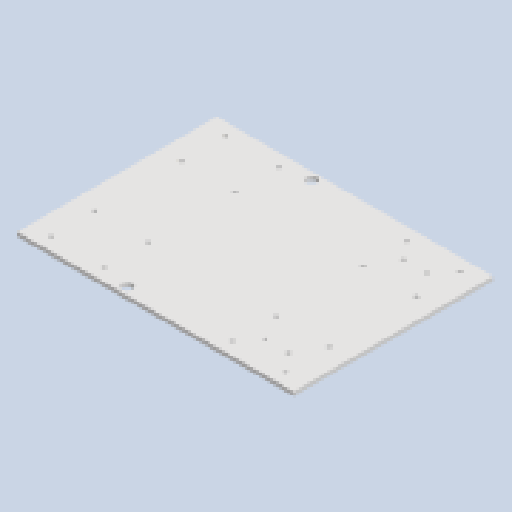
# Autodesk Inventor part: нижняя пластина
Saved by Autodesk Inventor 2024.2 (Build 282272000, 272)
## iProperties
Created: 2025-11-23
Part Number: нижняя пластина
Material: Типовые
Document SubType Name: Modeling
Designer: katya_notebook
Density: 1 g/cm^3
Appearance: По умолчанию
Author: katya_notebook
Autodesk Inventor part; units mm, degrees
ref_plane "YZ Plane" through (0, 0, 0) normal (1, 0, 0) x (0, 1, 0)
ref_plane "XZ Plane" through (0, 0, 0) normal (0, 1, 0) x (-1, 0, 0)
ref_plane "XY Plane" through (0, 0, 0) normal (0, 0, 1) x (1, 0, 0)
ref_plane "РабПлоскость1" through (-553.2789, -264.3002, 1.4222) normal (0, 1, 0) x (-1, 0, 0)
sketch "Эскиз1" plane through (-553.2789, -264.3002, 1.4222) normal (0, 1, 0) x (-1, 0, 0)
  line L0 (-30, 163.5) -> (30, 163.5) projected
  line L1 (-30, -31.5) -> (30, -31.5) projected
  line L2 (46.4763, 163.5) -> (-223.5237, 163.5)
  line L3 (-223.5237, 163.5) -> (-223.5237, -31.5)
  line L4 (-223.5237, -31.5) -> (46.4763, -31.5)
  line L5 (46.4763, -31.5) -> (46.4763, 163.5)
  point P0 (-553.2789, -1.4222)
  point P1 (-30, -30)
  point P2 (30, -30)
  point P3 (30, 162)
  point P4 (-30, 162)
  dimension "d1" = 270
  dimension "d6" = 0
  dimension "d7" = 0
  constraints: 8 end point, 2 coincident, 2 parallel, 1 horizontal, 1 perpendicular
  measures "d1" distance of L2.start L2.end
  measures "d6" distance from line of L4 L1.end
  measures "d7" distance from line of L2 L0.end
extrude "Выдавливание1" add sketch "Эскиз1" along normal blind 4
sketch "Эскиз2" plane through (-553.2789, -264.3002, 1.4222) normal (0, -1, 0) x (1, 0, 0)
  circle A0 centre (26, 108.5) radius 2 projected
  circle A1 centre (-26, 151) radius 2 projected
  circle A2 centre (26, 151) radius 2 projected
  circle A3 centre (-26, 108.5) radius 2 projected
  line L0 (-21.5, 122) -> (-21.5, 157) projected
  line L1 (-23.5, 122) -> (-21.5, 122) projected
  line L2 (-23.5, 157) -> (-23.5, 122) projected
  line L3 (-30, 157) -> (-23.5, 157) projected
  line L4 (-30, 157) -> (-30, 103.5) projected
  line L5 (-30, 103.5) -> (30, 103.5) projected
  line L6 (30, 103.5) -> (30, 157) projected
  line L7 (23.5, 157) -> (30, 157) projected
  line L8 (23.5, 122) -> (23.5, 157) projected
  line L9 (21.5, 122) -> (23.5, 122) projected
  line L10 (21.5, 157) -> (21.5, 122) projected
  line L11 (-21.5, 157) -> (21.5, 157) projected
  circle A4 centre (26, 23.5) radius 2 projected
  circle A5 centre (-26, -19) radius 2 projected
  circle A6 centre (26, -19) radius 2 projected
  circle A7 centre (-26, 23.5) radius 2 projected
  line L12 (-21.5, 10) -> (-21.5, -25) projected
  line L13 (-21.5, -25) -> (21.5, -25) projected
  line L14 (21.5, -25) -> (21.5, 10) projected
  line L15 (21.5, 10) -> (23.5, 10) projected
  line L16 (23.5, 10) -> (23.5, -25) projected
  line L17 (23.5, -25) -> (30, -25) projected
  line L18 (30, 28.5) -> (30, -25) projected
  line L19 (-30, 28.5) -> (30, 28.5) projected
  line L20 (-30, -25) -> (-30, 28.5) projected
  line L21 (-30, -25) -> (-23.5, -25) projected
  line L22 (-23.5, -25) -> (-23.5, 10) projected
  line L23 (-23.5, 10) -> (-21.5, 10) projected
  circle A8 centre (26, -19) radius 2
  circle A9 centre (26, 23.5) radius 2
  circle A10 centre (-26, -19) radius 2
  circle A11 centre (-26, 23.5) radius 2
  circle A12 centre (26, 108.5) radius 2
  circle A13 centre (26, 151) radius 2
  circle A14 centre (-26, 108.5) radius 2
  circle A15 centre (-26, 151) radius 2
  point P0 (553.2789, -1.4222)
  constraints: 8 centre point, 8 coincident, 8 concentric
extrude "Выдавливание2" cut sketch "Эскиз2" against normal blind 4 contours A0 | A1 | A2 | A3 | A4 | A5 | A6 | A7
sketch "Эскиз3" plane through (-553.2789, -264.3002, 1.4222) normal (0, -1, 0) x (1, 0, 0)
  spline S0 degree 3 poles (167.5306, -1.5) (167.5306, -1.6752) (167.5059, -1.8631) (167.407, -2.2163) (167.333, -2.3816) (167.1432, -2.702) (167.0026, -2.8694) (166.6948, -3.1391) (166.528, -3.2419) (165.9933, -3.4904) (165.5892, -3.534) (164.8487, -3.4171) (164.5121, -3.2574) (164.0242, -2.8457) (163.7999, -2.5683) (163.6284, -2.1264) (163.5929, -2.0111) (163.5438, -1.7621) (163.5306, -1.6279) (163.5306, -1.3721) (163.5438, -1.2379) (163.5929, -0.9889) (163.6284, -0.8736) (163.7999, -0.4317) (164.0242, -0.1543) (164.5121, 0.2574) (164.8487, 0.4171) (165.5892, 0.534) (165.9933, 0.4904) (166.528, 0.2419) (166.6948, 0.1391) (167.0026, -0.1306) (167.1432, -0.298) (167.333, -0.6184) (167.407, -0.7837) (167.5059, -1.1369) (167.5306, -1.3248) (167.5306, -1.5) knots -1.597181 -1.597181 -1.597181 -1.597181 -1.544613 -1.544613 -1.492044 -1.492044 -1.42258 -1.42258 -1.353115 -1.353115 -1.1824 -1.1824 -1.011685 -1.011685 -0.875329 -0.875329 -0.83696 -0.83696 -0.798591 -0.798591 -0.760221 -0.760221 -0.721852 -0.721852 -0.585496 -0.585496 -0.414781 -0.414781 -0.244066 -0.244066 -0.174601 -0.174601 -0.105137 -0.105137 -0.052568 -0.052568 0 0 0 0 projected
  spline S1 degree 3 poles (190.0475, -1.5) (190.0475, -1.6203) (190.0365, -1.7387) (189.9958, -1.9661) (189.9661, -2.0751) (189.8558, -2.3816) (189.7534, -2.5587) (189.3863, -3.0484) (189.0432, -3.2817) (188.267, -3.5292) (187.833, -3.5367) (187.2363, -3.3378) (187.0421, -3.2434) (186.6807, -2.9773) (186.5141, -2.805) (186.2864, -2.4643) (186.1972, -2.2855) (186.0776, -1.9002) (186.0475, -1.6935) (186.0475, -1.3065) (186.0776, -1.0998) (186.1972, -0.7145) (186.2864, -0.5357) (186.5141, -0.195) (186.6807, -0.0227) (187.0421, 0.2434) (187.2363, 0.3378) (187.833, 0.5367) (188.267, 0.5292) (189.0432, 0.2817) (189.3863, 0.0484) (189.7534, -0.4413) (189.8558, -0.6184) (189.9661, -0.9249) (189.9958, -1.0339) (190.0365, -1.2613) (190.0475, -1.3797) (190.0475, -1.5) knots -1.539921 -1.539921 -1.539921 -1.539921 -1.503835 -1.503835 -1.467748 -1.467748 -1.395575 -1.395575 -1.217174 -1.217174 -1.038772 -1.038772 -0.962412 -0.962412 -0.886052 -0.886052 -0.828007 -0.828007 -0.769961 -0.769961 -0.711915 -0.711915 -0.653869 -0.653869 -0.577509 -0.577509 -0.501149 -0.501149 -0.322747 -0.322747 -0.144346 -0.144346 -0.072173 -0.072173 -0.036086 -0.036086 0 0 0 0 projected
  circle A0 centre (203.0475, 23.5) radius 2 projected
  circle A1 centre (203.0475, -19) radius 2 projected
  circle A2 centre (151.0475, 23.5) radius 2 projected
  circle A3 centre (151.0475, -19) radius 2 projected
  line L0 (206.803, 28.5) -> (146.803, 28.5) projected
  line L1 (146.803, 28.5) -> (146.803, -25) projected
  line L2 (206.803, -25) -> (206.803, 28.5) projected
  line L3 (146.803, -25) -> (206.803, -25) projected
  point P0 (553.2789, -1.4222)
  point P1 (167.5306, -1.5)
  point P2 (190.0475, -1.5)
extrude "Выдавливание3" cut sketch "Эскиз3" against normal blind 10 contours S0 | S1 | A0 | A1 | A2 | A3
sketch "Эскиз4" plane through (-553.2789, -264.3002, 1.4222) normal (0, -1, 0) x (1, 0, 0)
  circle A0 centre (151.0475, 108.5) radius 2 projected
  circle A1 centre (203.0475, 108.5) radius 2 projected
  spline S0 degree 3 poles (190.0475, 133.5) (190.0475, 133.6203) (190.0365, 133.7387) (189.9958, 133.9661) (189.9661, 134.0751) (189.8558, 134.3816) (189.7534, 134.5587) (189.3863, 135.0484) (189.0432, 135.2817) (188.267, 135.5292) (187.833, 135.5367) (187.2363, 135.3378) (187.0421, 135.2435) (186.6807, 134.9773) (186.5141, 134.805) (186.2864, 134.4643) (186.1972, 134.2856) (186.0776, 133.9002) (186.0475, 133.6935) (186.0475, 133.3065) (186.0776, 133.0998) (186.1972, 132.7145) (186.2864, 132.5357) (186.5141, 132.195) (186.6807, 132.0227) (187.0421, 131.7566) (187.2363, 131.6622) (187.833, 131.4634) (188.267, 131.4708) (189.0432, 131.7183) (189.3863, 131.9517) (189.7534, 132.4413) (189.8558, 132.6184) (189.9661, 132.9249) (189.9958, 133.0339) (190.0365, 133.2613) (190.0475, 133.3797) (190.0475, 133.5) knots 0 0 0 0 0.036086 0.036086 0.072173 0.072173 0.144346 0.144346 0.322747 0.322747 0.501149 0.501149 0.577509 0.577509 0.653869 0.653869 0.711915 0.711915 0.769961 0.769961 0.828007 0.828007 0.886052 0.886052 0.962412 0.962412 1.038772 1.038772 1.217174 1.217174 1.395575 1.395575 1.467748 1.467748 1.503835 1.503835 1.539921 1.539921 1.539921 1.539921 projected
  spline S1 degree 3 poles (167.5306, 133.5) (167.5306, 133.6752) (167.5059, 133.8631) (167.407, 134.2163) (167.333, 134.3816) (167.1432, 134.702) (167.0026, 134.8694) (166.6948, 135.1391) (166.528, 135.2419) (165.9933, 135.4904) (165.5892, 135.534) (164.8487, 135.4171) (164.5121, 135.2574) (164.0242, 134.8457) (163.7999, 134.5683) (163.6284, 134.1264) (163.5929, 134.0111) (163.5438, 133.7621) (163.5306, 133.6279) (163.5306, 133.3721) (163.5438, 133.2379) (163.5929, 132.9889) (163.6284, 132.8736) (163.7999, 132.4317) (164.0242, 132.1543) (164.5121, 131.7426) (164.8487, 131.5829) (165.5892, 131.466) (165.9933, 131.5096) (166.528, 131.7581) (166.6948, 131.8609) (167.0026, 132.1306) (167.1432, 132.298) (167.333, 132.6184) (167.407, 132.7837) (167.5059, 133.1369) (167.5306, 133.3248) (167.5306, 133.5) knots 0 0 0 0 0.052568 0.052568 0.105137 0.105137 0.174601 0.174601 0.244066 0.244066 0.414781 0.414781 0.585496 0.585496 0.721852 0.721852 0.760221 0.760221 0.798591 0.798591 0.83696 0.83696 0.875329 0.875329 1.011685 1.011685 1.1824 1.1824 1.353115 1.353115 1.42258 1.42258 1.492044 1.492044 1.544613 1.544613 1.597181 1.597181 1.597181 1.597181 projected
  circle A2 centre (151.0475, 151) radius 2 projected
  circle A3 centre (203.0475, 151) radius 2 projected
  point P0 (553.2789, -1.4222)
  point P1 (190.0475, 133.5)
  point P2 (167.5306, 133.5)
extrude "Выдавливание4" cut sketch "Эскиз4" against normal blind 10
sketch "Эскиз6" plane through (-553.2789, -264.3002, 1.4222) normal (0, -1, 0) x (1, 0, 0)
  circle A0 centre (53.5237, 156) radius 5 projected
  circle A1 centre (53.5237, 156) radius 2.5 projected
  circle A2 centre (53.5237, 156) radius 5
  circle A3 centre (53.5237, -24) radius 5 projected
  circle A4 centre (53.5237, -24) radius 5
  point P0 (553.2789, -1.4222)
  constraints: 2 centre point, 2 coincident, 2 concentric
extrude "Выдавливание6" cut sketch "Эскиз6" against normal blind 10 contours A0 | A1 | A3
